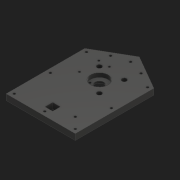
# Autodesk Inventor part: AC02
Saved by Autodesk Inventor 2017 (Build 210142000, 142)
## iProperties
Created: 2019-08-28
Part Number: AC02
Material: ABS Plastic
Document SubType Name: Modeling
Designer: Dell
Density: 1.06 g/cm^3
Appearance: Smooth - Black
Author: Dell
Autodesk Inventor part; units mm, degrees
ref_plane "YZ Plane" through (0, 0, 0) normal (1, 0, 0) x (0, 1, 0)
ref_plane "XZ Plane" through (0, 0, 0) normal (0, 1, 0) x (-1, 0, 0)
ref_plane "XY Plane" through (0, 0, 0) normal (0, 0, 1) x (1, 0, 0)
sketch "Sketch35" plane through (0, 0, 0) normal (0, 0, 1) x (1, 0, 0)
  line L0 (0, 68.1273) -> (59, 34.0637)
  line L1 (59, 34.0637) -> (59, -34.0637)
  line L2 (59, -34.0637) -> (0, -68.1273)
  line L3 (0, -68.1273) -> (-59, -34.0637)
  line L4 (-59, -34.0637) -> (-59, 34.0637)
  line L5 (-59, 34.0637) -> (0, 68.1273)
  line L6 (-59, -34.0637) -> (-59, -100)
  line L7 (-59, -100) -> (59, -100)
  line L8 (59, -100) -> (59, -34.0637)
  point P0 (0, 0)
  point P1 (0, 0)
  dimension "d165" = 118
  dimension "d166" = 100
  constraints: 18 end point, 2 perpendicular, 1 coincident, 1 vertical, 1 vertical alignment, 13 other
  measures "d165" distance between parallel lines of L1 L4
  measures "d166" distance from line of L7 point (0, 0)
extrude "Extrusion34" add sketch "Sketch35" along normal blind 55
sketch "Sketch36" plane through (0, 0, 55) normal (0, 0, 1) x (1, 0, 0)
  line L0 (59, -100) -> (59, 34.0637) construction
  line L1 (59, 34.0637) -> (0, 68.1273) construction
  line L2 (0, 68.1273) -> (-59, 34.0637) construction
  line L3 (-59, 34.0637) -> (-59, -100) construction
  line L4 (-59, -100) -> (59, -100) construction
  line L5 (52, 30.0222) -> (52, -93) construction
  line L6 (52, -93) -> (-52, -93) construction
  line L7 (-52, -93) -> (-52, 30.0222) construction
  line L8 (-52, 30.0222) -> (0, 60.0444) construction
  line L9 (0, 60.0444) -> (52, 30.0222) construction
  circle A0 centre (-52, -93) radius 2
  circle A1 centre (52, -93) radius 2
  circle A2 centre (0, 60.0444) radius 2
  circle A3 centre (-52, 30.0222) radius 2
  circle A4 centre (52, 30.0222) radius 2
  circle A5 centre (-26, -93) radius 2
  circle A6 centre (26, -93) radius 2
  circle A7 centre (0, -93) radius 2
  circle A8 centre (-52, -61.4889) radius 2
  circle A9 centre (-52, -31.4889) radius 2
  circle A10 centre (-52, 0) radius 2
  circle A11 centre (52, 0) radius 2
  circle A12 centre (52, -31.4889) radius 2
  circle A13 centre (52, -61.4889) radius 2
  circle A14 centre (-26, 45.0333) radius 2
  circle A15 centre (26, 45.0333) radius 2
  point P0 (0, 0)
  dimension "d169" = 7
  dimension "d170" = 4
  dimension "d171" = 4
  dimension "d172" = 4
  dimension "d173" = 4
  dimension "d174" = 4
  dimension "d175" = 4
  dimension "d176" = 4
  dimension "d177" = 4
  dimension "d178" = 4
  dimension "d179" = 4
  dimension "d180" = 4
  dimension "d181" = 4
  dimension "d182" = 4
  dimension "d183" = 4
  dimension "d184" = 4
  dimension "d185" = 4
  dimension "d186" = 30
  constraints: 16 centre point, 10 end point, 6 point on line, 5 coincident, 5 midpoint, 3 horizontal alignment, 2 vertical alignment, 4 other
  measures "d169" distance between parallel lines of L0 L5
  measures "d170" diameter of A0
  measures "d171" diameter of A1
  measures "d172" diameter of A2
  measures "d173" diameter of A3
  measures "d174" diameter of A4
  measures "d175" diameter of A5
  measures "d176" diameter of A6
  measures "d177" diameter of A7
  measures "d178" diameter of A8
  measures "d179" diameter of A9
  measures "d180" diameter of A10
  measures "d181" diameter of A11
  measures "d182" diameter of A12
  measures "d183" diameter of A13
  measures "d184" diameter of A14
  measures "d185" diameter of A15
  measures "d186" distance of A9.centre A8.centre
extrude "Extrusion35" cut sketch "Sketch36" against normal through all contours A0 | A1 | A3 | A4 | A7 | A9 | A12 | A14 | A15
sketch "Sketch37" plane through (0, 0, 55) normal (0, 0, 1) x (1, 0, 0)
  circle A0 centre (0, 0) radius 15
  dimension "d189" = 30
  constraints: 1 centre point, 1 coincident
  measures "d189" diameter of A0
extrude "Extrusion36" cut sketch "Sketch37" against normal blind 7
sketch "Sketch41" plane through (0, 0, 0) normal (0, 0, -1) x (-1, 0, 0)
  circle A0 centre (26, 45.0333) radius 2 projected
  circle A1 centre (-52, -31.4889) radius 2 projected
  circle A2 centre (-52, 30.0222) radius 2 projected
  circle A3 centre (52, -93) radius 2 projected
  circle A4 centre (-52, -93) radius 2 projected
  circle A5 centre (52, 30.0222) radius 2 projected
  circle A6 centre (0, -93) radius 2 projected
  circle A7 centre (52, -31.4889) radius 2 projected
  circle A8 centre (-26, 45.0333) radius 2 projected
  line L0 (-59, -100) -> (-59, 34.0637) projected
  line L1 (59, -100) -> (-59, -100) projected
  line L2 (59, 34.0637) -> (59, -100) projected
  line L3 (0, 68.1273) -> (59, 34.0637) projected
  line L4 (-59, 34.0637) -> (0, 68.1273) projected
  line L5 (0, 51.9615) -> (45, 25.9808)
  line L6 (45, 25.9808) -> (45, -86)
  line L7 (45, -86) -> (-45, -86)
  line L8 (-45, -86) -> (-45, 25.9808)
  line L9 (-45, 25.9808) -> (0, 51.9615)
  point P0 (0, 0)
  dimension "d199" = 14
  constraints: 10 end point, 4 other
  measures "d199" distance between parallel lines of L8 L0
extrude "Extrusion39" cut sketch "Sketch41" against normal blind 45 contours L0 L4 L3 L2 L1 | L5 L6 L7 L8 L9
sketch "Sketch42" plane through (0, 0, 45) normal (0, 0, -1) x (-1, 0, 0)
  circle A0 centre (0, 0) radius 7.5
  circle A1 centre (-19.799, -19.799) radius 4
  circle A2 centre (-21.2132, 21.2132) radius 4
  circle A3 centre (19.799, 19.799) radius 4
  line L0 (0, 0) -> (32.276, 0) construction
  line L1 (0, 0) -> (-19.799, -19.799) construction
  line L2 (0, 0) -> (-21.2132, 21.2132) construction
  line L3 (0, 0) -> (19.799, 19.799) construction
  line L4 (10.799, 27.799) -> (28.799, 27.799) construction
  line L5 (28.799, 27.799) -> (28.799, -5.201) construction
  line L6 (28.799, -5.201) -> (10.799, -5.201) construction
  line L7 (10.799, -5.201) -> (10.799, 27.799) construction
  circle A4 centre (10.799, 27.799) radius 1.75
  circle A5 centre (28.799, 27.799) radius 1.75
  circle A6 centre (28.799, -5.201) radius 1.75
  circle A7 centre (10.799, -5.201) radius 1.75
  point P0 (19.799, 27.799)
  dimension "d202" = 15
  dimension "d203" = 8
  dimension "d204" = 8
  dimension "d205" = 8
  dimension "d206" = 28
  dimension "d207" = 30
  dimension "d208" = 28
  dimension "d209" = 45
  dimension "d210" = 18
  dimension "d211" = 33
  dimension "d212" = 8
  dimension "d213" = 3.5
  dimension "d214" = 3.5
  dimension "d215" = 3.5
  dimension "d216" = 3.5
  dimension "d219" = 135
  dimension "d220" = 135
  constraints: 16 end point, 8 centre point, 5 coincident, 2 horizontal, 2 parallel, 1 midpoint, 1 perpendicular, 1 vertical alignment
  measures "d202" diameter of A0
  measures "d203" diameter of A1
  measures "d204" diameter of A2
  measures "d205" diameter of A3
  measures "d206" distance of point (0, 0) L3.end
  measures "d207" distance of point (0, 0) L2.end
  measures "d208" distance of point (0, 0) L1.end
  measures "d209" angle of L0 L3
  measures "d210" distance of L4.start L4.end
  measures "d211" distance of L4.end L5.end
  measures "d212" distance from line of L4 L3.end
  measures "d213" diameter of A4
  measures "d214" diameter of A5
  measures "d215" diameter of A6
  measures "d216" diameter of A7
  measures "d219" angle of L0 L1
  measures "d220" angle of L2 L0
extrude "Extrusion40" cut sketch "Sketch42" against normal through all
sketch "Sketch43" plane through (0, 0, 45) normal (0, 0, -1) x (-1, 0, 0)
  line L0 (-6.5, -73) -> (6.5, -73)
  line L1 (6.5, -73) -> (6.5, -86)
  line L2 (6.5, -86) -> (-6.5, -86)
  line L3 (-6.5, -86) -> (-6.5, -73)
  line L4 (59, -100) -> (-59, -100) projected
  point P0 (0, 0)
  point P1 (0, -73)
  dimension "d221" = 13
  dimension "d222" = 13
  dimension "d223" = 27
  constraints: 8 end point, 2 parallel, 1 horizontal, 1 midpoint, 1 perpendicular, 1 vertical alignment
  measures "d221" distance of L1.end L2.end
  measures "d222" distance of L0.end L1.end
  measures "d223" distance between parallel lines of L4 L0
extrude "Extrusion41" cut sketch "Sketch43" against normal through all
sketch "Sketch44" plane through (0, 0, 45) normal (0, 0, -1) x (-1, 0, 0)
  circle A0 centre (0, 53.1273) radius 2
  circle A1 centre (-34, -75) radius 2
  line L0 (-59, -100) -> (-59, 34.0637) projected
  line L1 (59, -100) -> (-59, -100) projected
  point P0 (0, 0)
  point P1 (0, 68.1273)
  dimension "d226" = 4
  dimension "d227" = 4
  dimension "d228" = 15
  dimension "d229" = 25
  dimension "d230" = 25
  constraints: 2 centre point, 1 vertical alignment
  measures "d226" diameter of A0
  measures "d227" diameter of A1
  measures "d228" distance of point (0, 68.127) A0.centre
  measures "d229" distance from line of L0 A1.centre
  measures "d230" distance from line of L1 A1.centre
extrude "Extrusion42" cut sketch "Sketch44" against normal through all
sketch "Sketch45" plane through (0, 0, 45) normal (0, 0, -1) x (-1, 0, 0)
  circle A0 centre (19.799, 19.799) radius 4 projected
  circle A1 centre (10.799, 27.799) radius 1.75 projected
  circle A2 centre (28.799, 27.799) radius 1.75 projected
  circle A3 centre (28.799, -5.201) radius 1.75 projected
  circle A4 centre (10.799, -5.201) radius 1.75 projected
  circle A5 centre (10.799, -5.201) radius 4.5
  circle A6 centre (10.799, 27.799) radius 7.5
  circle A7 centre (19.799, 19.799) radius 9
  circle A8 centre (28.799, 27.799) radius 1.75 projected
  circle A9 centre (28.799, 27.799) radius 7.5
  circle A10 centre (28.799, -5.201) radius 7.5
  point P0 (0, 0)
  dimension "d233" = 9
  dimension "d234" = 15
  dimension "d235" = 18
  dimension "d236" = 15
  dimension "d237" = 15
  constraints: 5 centre point, 5 coincident
  measures "d233" diameter of A5
  measures "d234" diameter of A6
  measures "d235" diameter of A7
  measures "d236" diameter of A9
  measures "d237" diameter of A10
extrude "Extrusion43" add sketch "Sketch45" along normal blind 4
equation "\"d213\" = d215"
equation "\"d214\" = d215"
equation "\"d216\" = d215"
body "Solid2"
